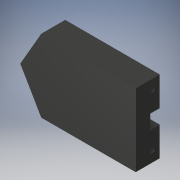
# Autodesk Inventor part: TARM06
Saved by Autodesk Inventor 2017 (Build 210142000, 142)
## iProperties
Created: 2018-10-19
Part Number: TARM06
Material: ABS Plastic
Document SubType Name: Modeling
Designer: Dell
Density: 1.06 g/cm^3
Appearance: Smooth - Black
Author: Dell
Autodesk Inventor part; units mm, degrees
ref_plane "YZ Plane" through (0, 0, 0) normal (1, 0, 0) x (0, 1, 0)
ref_plane "XZ Plane" through (0, 0, 0) normal (0, 1, 0) x (-1, 0, 0)
ref_plane "XY Plane" through (0, 0, 0) normal (0, 0, 1) x (1, 0, 0)
sketch "Sketch1" plane through (0, 0, 0) normal (0, 0, 1) x (1, 0, 0)
  line L0 (44.453, 0) -> (22.2265, -38.4974)
  line L1 (22.2265, -38.4974) -> (-22.2265, -38.4974)
  line L2 (-22.2265, -38.4974) -> (-44.453, 0)
  line L3 (-44.453, 0) -> (-22.2265, 38.4974)
  line L4 (-22.2265, 38.4974) -> (22.2265, 38.4974)
  line L5 (22.2265, 38.4974) -> (44.453, 0)
  line L6 (22.2265, 38.4974) -> (77.5, 38.4974)
  line L7 (22.2265, -38.4974) -> (77.5, -38.4974)
  line L8 (77.5, -38.4974) -> (77.5, 38.4974)
  point P0 (0, 0)
  point P1 (0, 0)
  dimension "d1" = 99.7265
  dimension "d2" = 76.9948
  constraints: 18 end point, 1 coincident, 1 horizontal, 1 horizontal alignment, 1 perpendicular, 1 point on line, 13 other
  measures "d1" distance of L6.end L3.end
  measures "d2" distance of L7.end L6.end
extrude "Extrusion1" add sketch "Sketch1" along normal blind 15
sketch "Sketch2" plane through (77.5, -38.4974, 0) normal (1, 0, 0) x (0, 0, -1)
  circle A0 centre (-7.5, 65.9974) radius 2.5
  circle A1 centre (-7.5, 10.9974) radius 2.5
  line L0 (-7.5, 65.9974) -> (-7.5, 10.9974) construction
  line L1 (0, 0) -> (0, 76.9948) construction
  line L2 (0, 76.9948) -> (-15, 76.9948) construction
  point P0 (0, 38.4974)
  point P1 (-7.5, 38.4974)
  point P2 (0, 38.4974)
  point P3 (-7.5, 76.9948)
  dimension "d5" = 5
  dimension "d6" = 5
  dimension "d7" = 55
  constraints: 3 midpoint, 2 centre point, 2 end point, 1 horizontal alignment, 1 vertical, 1 vertical alignment
  measures "d5" diameter of A0
  measures "d6" diameter of A1
  measures "d7" distance of L0.start L0.end
extrude "Extrusion2" cut sketch "Sketch2" against normal blind 25
sketch "Sketch3" plane through (0, 0, 0) normal (0, 0, -1) x (-1, 0, 0)
  line L0 (-77.5, -38.4974) -> (-77.5, 38.4974) projected
  line L1 (-77.5, 7.5) -> (-62.5, 7.5)
  line L2 (-62.5, 7.5) -> (-62.5, -7.5)
  line L3 (-62.5, -7.5) -> (-77.5, -7.5)
  line L4 (-77.5, -7.5) -> (-77.5, 7.5)
  line L5 (-77.5, 38.4974) -> (22.2265, 38.4974) projected
  line L6 (22.2265, 38.4974) -> (44.453, 0) projected
  line L7 (44.453, 0) -> (22.2265, -38.4974) projected
  line L8 (22.2265, -38.4974) -> (-77.5, -38.4974) projected
  line L9 (38.6795, 0) -> (19.3397, 33.4974)
  line L10 (19.3397, 33.4974) -> (-72.5, 33.4974)
  line L11 (-72.5, 33.4974) -> (-72.5, -33.4974) construction
  line L12 (-72.5, -33.4974) -> (19.3397, -33.4974)
  line L13 (19.3397, -33.4974) -> (38.6795, 0)
  line L14 (-62.5, 7.5) -> (-62.5, 33.4974)
  line L15 (-62.5, -7.5) -> (-62.5, -33.4974)
  line L16 (19.3397, 33.4974) -> (-62.5, 33.4974)
  line L17 (-62.5, -33.4974) -> (19.3397, -33.4974)
  point P0 (0, 0)
  point P1 (-77.5, 0)
  dimension "d10" = 15
  dimension "d11" = 15
  dimension "d12" = 5
  constraints: 26 end point, 4 point on line, 2 horizontal, 2 midpoint, 2 parallel, 2 perpendicular, 1 collinear, 4 other
  measures "d10" distance between parallel lines of L1 L3
  measures "d11" distance of L2.end L3.end
  measures "d12" distance between parallel lines of L6 L9
extrude "Extrusion3" cut sketch "Sketch3" against normal blind 10 contours L0 L1 L2 L3 | L2 L14 L10 L9 L13 L12 L15
sketch "Sketch5" plane through (0, 0, 15) normal (0, 0, 1) x (1, 0, 0)
  line L0 (77.5, 38.4974) -> (-22.2265, 38.4974) projected
  line L1 (-22.2265, 38.4974) -> (-44.453, 0) projected
  line L2 (-44.453, 0) -> (-22.2265, -38.4974) projected
  line L3 (-22.2265, -38.4974) -> (77.5, -38.4974) projected
  line L4 (77.5, -38.4974) -> (77.5, 38.4974) projected
  line L5 (77, -37.9974) -> (-21.9378, -37.9974)
  line L6 (-21.9378, -37.9974) -> (-43.8756, 0)
  line L7 (-43.8756, 0) -> (-21.9378, 37.9974)
  line L8 (-21.9378, 37.9974) -> (77, 37.9974)
  line L9 (77, 37.9974) -> (77, -37.9974)
  point P0 (0, 0)
  dimension "d15" = 0.5
  constraints: 10 end point, 4 other
  measures "d15" distance between parallel lines of L3 L5
extrude "Extrusion4" cut sketch "Sketch5" against normal through all
sketch "Sketch6" plane through (0, 0, 15) normal (0, 0, 1) x (1, 0, 0)
  line L0 (77, -37.9974) -> (77, 37.9974) projected
  line L1 (77, 37.9974) -> (-21.9378, 37.9974) projected
  line L2 (-21.9378, 37.9974) -> (-43.8756, 0) projected
  line L3 (-43.8756, 0) -> (-21.9378, -37.9974) projected
  line L4 (-21.9378, -37.9974) -> (77, -37.9974) projected
  point P0 (0, 0)
extrude "Extrusion5" add sketch "Sketch6" along normal blind 10
sketch "Sketch7" plane through (0, 0, 10) normal (0, 0, -1) x (-1, 0, 0)
  line L0 (-77, 7.5) -> (-77, -7.5) projected
  line L1 (-62.5, -7.5) -> (-77, -7.5) projected
  line L2 (-62.5, -27.5) -> (-62.5, -7.5) projected
  line L3 (-62.5, -33.4974) -> (-62.5, -27.5) projected
  line L4 (19.3397, -33.4974) -> (-62.5, -33.4974) projected
  line L5 (38.6795, 0) -> (19.3397, -33.4974) projected
  line L6 (19.3397, 33.4974) -> (38.6795, 0) projected
  line L7 (-62.5, 33.4974) -> (19.3397, 33.4974) projected
  line L8 (-62.5, 27.5) -> (-62.5, 33.4974) projected
  line L9 (-62.5, 7.5) -> (-62.5, 27.5) projected
  line L10 (-77, 7.5) -> (-62.5, 7.5) projected
  line L11 (-62.5, 7.5) -> (-62.5, -7.5)
  point P0 (0, 0)
  constraints: 2 end point, 1 vertical
extrude "Extrusion6" cut sketch "Sketch7" against normal blind 10 contours L9 L8 L7 L6 L5 L4 L3 L2 L11
body "Solid1"
